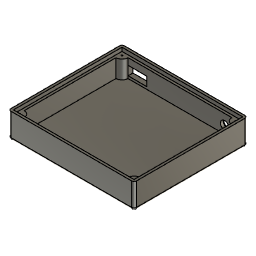
Case - Boden v6 (Autodesk Fusion 360 design; units mm, degrees)
Autodesk Fusion 360 part; units mm, degrees
note: some values were not read from the file. Set by a fixed rule: which sketch regions a step uses.
sketch "Skizze1" plane through (0, 0, 0) normal (0, 0, 1) x (1, 0, 0)
  line L0 (0, 0) -> (100, 0)
  line L1 (100, 0) -> (100, 90)
  line L2 (100, 90) -> (0, 90)
  line L3 (0, 90) -> (0, 0)
  dimension "d29" = 100
  dimension "d30" = 90
  constraint horizontal L0
  constraint vertical L1
  constraint horizontal L2
  constraint vertical L3
  constraint coincident L0.start L3.end
  measures "d29" distance of L0.start L0.end
  measures "d30" distance of L0.start L2.end
extrude "Extrusion1" add sketch "Skizze1" along normal blind 3 makes body 1
sketch "Skizze2" plane through (0, 0, 0) normal (0, 0, 1) x (1, 0, 0)
  line L0 (7, 2) -> (93, 2)
  line L1 (98, 7) -> (98, 83)
  line L2 (93, 88) -> (7, 88)
  line L3 (2, 83) -> (2, 7)
  arc A0 (7, 2) -> (2, 7) centre (2, 2) ccw
  arc A1 (2, 83) -> (7, 88) centre (2, 88) ccw
  arc A2 (93, 88) -> (98, 83) centre (98, 88) ccw
  arc A3 (98, 7) -> (93, 2) centre (98, 2) ccw
  dimension "d19" = 86
  dimension "d20" = 96
  dimension "d21" = 5
  dimension "d22" = 5
  dimension "d23" = 5
  dimension "d24" = 5
  dimension "d27" = 2
  dimension "d28" = 2
  constraint horizontal L0
  constraint vertical L1
  constraint horizontal L2
  constraint vertical L3
  measures "d19" distance of A0.centre A1.centre
  measures "d20" distance of A0.centre A3.centre
  measures "d21" radius of A1
  measures "d22" radius of A2
  measures "d23" radius of A3
  measures "d24" radius of A0
  measures "d27" horizontal distance of origin A0.centre
  measures "d28" vertical distance of origin A0.centre
extrude "Extrusion2" add sketch "Skizze2" against normal blind 15 bodies 1
sketch "Skizze3" plane through (0, 0, 0) normal (0, 0, 1) x (1, 0, 0)
  line L0 (-2, -2) -> (102, -2)
  line L1 (102, -2) -> (102, 92)
  line L2 (102, 92) -> (-2, 92)
  line L3 (-2, 92) -> (-2, -2)
  dimension "d5" = 104
  dimension "d6" = 94
  dimension "d25" = 2
  dimension "d26" = 2
  constraint horizontal L0
  constraint vertical L1
  constraint horizontal L2
  constraint vertical L3
  measures "d5" distance of L0.start L0.end
  measures "d6" distance of L0.start L2.end
  measures "d25" distance of origin L3
  measures "d26" distance of origin L0
extrude "Extrusion4" add sketch "Skizze3" along normal blind 3 and the other way blind 18 separate body makes body 2
fillet "Abrundung2" radius 2 8 edges at (-2, -2, -7.5) (50, -2, -18) (-2, 45, -18) (-2, 92, -7.5) (102, -2, -7.5) (102, 92, -7.5) (50, 92, -18) (102, 45, -18) on bodies 2
combine "Kombinieren1" operation cut target body 2 tool bodies 1 keep tools result as body 3 in component "Component"
sketch "Skizze5" plane through (0, 0, 0) normal (0, 0, 1) x (-1, 0, 0)
  arc A0 (-2, -83) -> (-7, -88) centre (-2, -88) ccw
  line L0 (-7, -88) -> (-93, -88)
  arc A1 (-93, -88) -> (-98, -83) centre (-98, -88) ccw
  line L1 (-98, -83) -> (-98, -7)
  arc A2 (-98, -7) -> (-93, -2) centre (-98, -2) ccw
  line L2 (-93, -2) -> (-7, -2)
  arc A3 (-7, -2) -> (-2, -7) centre (-2, -2) ccw
  line L3 (-2, -7) -> (-2, -83)
  line L4 (0, -90) -> (0, 0)
  line L5 (0, 0) -> (-100, 0)
  line L6 (-100, 0) -> (-100, -90)
  line L7 (-100, -90) -> (0, -90)
  line L8 (0, 0) -> (-5.5355, -5.5355)
  circle A4 centre (-2.7678, -2.7678) radius 0.5 construction
  line L9 (0, -90) -> (-5.5355, -84.4645)
  line L10 (-100, -90) -> (-94.4645, -84.4645)
  line L11 (-100, 0) -> (-94.4645, -5.5355)
  point P0 (-2.9019, -87.0981)
  point P1 (-97.2322, -87.2322)
  point P2 (-97.2322, -2.7678)
  dimension "d31" = 1
  constraint coincident L4.end L5.start
  constraint midpoint A3 L8.end
  constraint coincident L8 A4.centre
  constraint midpoint L8 A4.centre
  constraint coincident L4.start L7.end
  constraint midpoint A0 L9.end
  constraint coincident L9 P0
  constraint coincident L6.end L7.start
  constraint midpoint A1 L10.end
  constraint midpoint L10 P1
  constraint coincident L5.end L6.start
  constraint midpoint A2 L11.end
  constraint midpoint L11 P2
  measures "d31" diameter of A4
hole "Bohrung1" at (2.7678, 2.7678, 0) direction (0, 0, -1) diameter 1.2 depth 6 tip angle 118 bodies 3 in component "Component"
hole "Bohrung2" at (2.9019, 87.0981, 0) direction (0, 0, -1) diameter 1.2 depth 6 tip angle 118 bodies 3 in component "Component"
hole "Bohrung3" at (97.2322, 2.7678, 0) direction (0, 0, -1) diameter 1.2 depth 6 tip angle 118 bodies 3 in component "Component"
hole "Bohrung4" at (97.2322, 87.2322, 0) direction (0, 0, -1) diameter 1.2 depth 6 tip angle 118 bodies 3 in component "Component"
hole "pwr con" at (87.1068, 92, -8.5471) direction (0, -1, 0) diameter 7 depth 4 tip angle 180 counterbore diameter 10 counterbore depth 1.6 bodies 3 in component "Component"
sketch "Skizze6" plane through (0, 92, 0) normal (0, 1, 0) x (-1, 0, 0)
  circle A0 centre (-87.1068, -8.5471) radius 5
  line L0 (-100, 3) -> (-100, -16)
  line L1 (-100, -16) -> (0, -16)
  line L2 (0, -16) -> (0, 3)
  line L3 (0, 3) -> (-100, 3)
  line L4 (-7, -13) -> (-22.5, -13)
  line L5 (-22.5, -13) -> (-22.5, -5.5)
  line L6 (-22.5, -5.5) -> (-7, -5.5)
  line L7 (-7, -5.5) -> (-7, -13)
  line L8 (2, 3) -> (2, -16)
  line L9 (0, -18) -> (-100, -18)
  dimension "d54" = 15.5
  dimension "d55" = 7.5
  dimension "d56" = 9
  dimension "d57" = 5
  constraint vertical L5
  constraint horizontal L6
  measures "d54" distance of L5.end L6.end
  measures "d55" distance of L4.end L5.end
  measures "d56" distance of L6.end L8
  measures "d57" distance of L4.start L9
extrude "pwr switch loch" cut sketch "Skizze6" against normal blind 4 contours L4 L5 L6 L7 bodies 3 in component "Component"
component "Component" placed x (1, 0, 0) y (0, 1, 0) z (0, 0, 1) at (0, 0, 0)
named bodies: "Negativ", "case"
